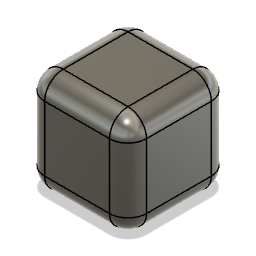
Cubo v8 (Autodesk Fusion 360 design; units mm, degrees)
Autodesk Fusion 360 part; units mm, degrees
sketch "Schizzo1" plane through (0, 0, 0) normal (0, 1, 0) x (1, 0, 0)
  line L0 (0, 0) -> (-11, 0)
  line L1 (-11, 0) -> (-11, -11)
  line L2 (-11, -11) -> (0, -11)
  line L3 (0, -11) -> (0, 0)
  dimension "d3" = 11
  dimension "d4" = 11
  constraint horizontal L0
  constraint vertical L1
  constraint horizontal L2
  constraint vertical L3
  constraint coincident L0.start L3.end
  measures "d3" distance of L0.start L0.end
  measures "d4" distance of L0.start L2.end
extrude "Estrusione1" add sketch "Schizzo1" along normal blind 11
fillet "Raccordo1" radius 2 12 edges at (-5.5, 11, 11) (0, 11, 5.5) (-11, 11, 5.5) (-5.5, 11, 0) (-11, 5.5, 0) (-11, 0, 5.5) (-11, 5.5, 11) (-5.5, 0, 11) (0, 0, 5.5) (-5.5, 0, 0) (0, 5.5, 0) (0, 5.5, 11)
